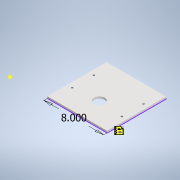
# Autodesk Inventor part: base_plate
Saved by Autodesk Inventor 2022 (Build 260153000, 153)
## iProperties
Created: 2021-10-26
Part Number: base_plate
Material: Generic
Document SubType Name: Modeling
Designer: pauly
Density: 1 g/cm^3
Appearance: Default
Author: pauly
Autodesk Inventor part; units mm, degrees
ref_plane "YZ Plane" through (0, 0, 0) normal (1, 0, 0) x (0, 1, 0)
ref_plane "XZ Plane" through (0, 0, 0) normal (0, 1, 0) x (-1, 0, 0)
ref_plane "XY Plane" through (0, 0, 0) normal (0, 0, 1) x (1, 0, 0)
sketch "Sketch1" plane through (0, 0, 0) normal (0, 1, 0) x (-1, 0, 0)
  line L0 (-330.2, -201.9268) -> (-330.2, 0)
  line L1 (-127, -201.9268) -> (-330.2, -201.9268)
  line L2 (-330.2, 0) -> (-127, 0)
  line L3 (-127, 0) -> (-127, -201.9268)
  point P0 (0, 0)
  dimension "d136" = 203.2
  constraints: 8 end point, 2 perpendicular
  measures "d136" distance of L2.end L0.end
extrude "Extrusion1" add sketch "Sketch1" along normal blind 6.35
sketch "Sketch2" plane through (0, 6.35, 0) normal (0, 1, 0) x (1, 0, 0)
  circle A0 centre (143.9333, 141.1986) radius 2.6501
  circle A1 centre (143.9333, 67.4878) radius 2.6501
  circle A2 centre (313.2667, 141.1986) radius 2.6501
  circle A3 centre (313.2667, 67.4878) radius 2.6501
  line L0 (330.2, 0) -> (127, 0)
  line L1 (127, 0) -> (330.2, 0) projected
  line L2 (330.2, 0) -> (330.2, 201.9268) projected
  line L3 (330.2, 0) -> (330.2, 201.9268)
  line L4 (330.2, 201.9268) -> (127, 201.9268)
  line L5 (127, 201.9268) -> (127, 0) projected
  line L6 (127, 201.9268) -> (127, 0)
  point P0 (127, 19.4733)
  point P1 (330.2, 149.86)
  point P2 (228.6, 0)
  dimension "d137" = 203.2
  constraints: 8 end point, 4 centre point, 2 perpendicular, 1 midpoint, 1 vertical
  measures "d137" distance of L0.start L0.end
hole "Hole9" at (143.9333, 6.35, -141.1986) direction (0, -1, 0) diameter 6.4008 end through all thread size "5/16-18 UNC" class "2B" standard "ANSI Unified Screw Threads"
hole "Hole10" at (143.9333, 6.35, -67.4878) direction (0, -1, 0) diameter 6.4008 end through all thread size "5/16-18 UNC" class "2B" standard "ANSI Unified Screw Threads"
hole "Hole11" at (313.2667, 6.35, -141.1986) direction (0, -1, 0) diameter 6.4008 end through all thread size "5/16-18 UNC" class "2B" standard "ANSI Unified Screw Threads"
hole "Hole12" at (313.2667, 6.35, -67.4878) direction (0, -1, 0) diameter 6.4008 end through all thread size "5/16-18 UNC" class "2B" standard "ANSI Unified Screw Threads"
sketch "Sketch3" plane through (0, 6.35, 0) normal (0, 1, 0) x (1, 0, 0)
  circle A0 centre (228.6, 75.5634) radius 17.9959
  point P0 (0, 0)
  point P1 (127, 201.9268)
  constraints: 1 centre point
extrude "Extrusion2" cut sketch "Sketch3" against normal blind 50.8
equation "\"d97\" = d12"
equation "\"d104\" = d12"
equation "\"d111\" = d12"
equation "\"d12\" = 7.9375"
body "Solid1"
